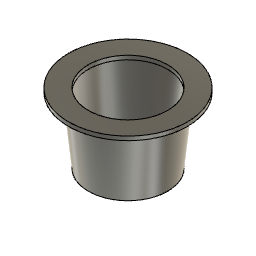
strong plant pot (Autodesk Fusion 360 design; units mm, degrees)
Autodesk Fusion 360 part; units mm, degrees
sketch "Sketch1" plane through (0, 0, 0) normal (0, 0, 1) x (1, 0, 0)
  circle A0 centre (0, 0) radius 30
  circle A1 centre (0, 0) radius 25
  dimension "d1" = 60
  dimension "d7" = 50
  constraint coincident A0.centre A1.centre
  constraint concentric A0 A1
  measures "d1" diameter of A0
  measures "d7" diameter of A1
ref_plane "WorkPlane1" through (0, 0, 50) normal (0, 0, 1) x (1, 0, 0)
ref_plane "WorkPlane2" through (0, 0, 50) normal (0, 0, 1) x (1, 0, 0)
ref_plane "WorkPlane3" through (0, 0, 50) normal (0, 0, 1) x (1, 0, 0)
sketch "Sketch7" plane through (0, 0, 50) normal (0, 0, 1) x (1, 0, 0)
  circle A0 centre (0, 0) radius 35
  circle A1 centre (0, 0) radius 30
  dimension "d6" = 70
  dimension "d8" = 60
  constraint coincident A0.centre A1.centre
  measures "d6" diameter of A0
  measures "d8" diameter of A1
loft "Loft1" add profiles "Sketch7", "Sketch1" section 1 section 2
sketch "Sketch8" plane through (0, 0, 50) normal (0, 0, 1) x (-1, 0, 0)
  circle A0 centre (0, 0) radius 35
  circle A1 centre (0, 0) radius 30
  dimension "d9" = 60
  constraint coincident A0.centre A1.centre
  measures "d9" diameter of A1
sketch "Sketch9" plane through (0, 0, 0) normal (0, 0, -1) x (1, 0, 0)
  circle A0 centre (0, 0) radius 30
  circle A1 centre (0, 0) radius 25
  constraint coincident A0.centre A1.centre
loft "Loft2" cut profiles "Sketch8", "Sketch9" section 1 contours A1 section 2 contours A1
sketch "Sketch11" plane through (0, 0, 50) normal (0, 0, 1) x (-1, 0, 0)
  circle A0 centre (0, 0) radius 30
  circle A1 centre (0, 0) radius 35
  circle A2 centre (0, 0) radius 30
  circle A3 centre (0, 0) radius 45
  dimension "d14" = 90
  constraint coincident A0.centre A1.centre
  constraint concentric A2 A3
  measures "d14" diameter of A3
extrude "Extrude2" add sketch "Sketch11" along normal blind 3 contours A1 | A3
sketch "Sketch12" plane through (0, 0, 0) normal (0, 0, -1) x (1, 0, 0)
  circle A0 centre (0, 0) radius 25
  circle A1 centre (0, 0) radius 30
  circle A2 centre (0, 0) radius 25
  circle A3 centre (0, 0) radius 20
  dimension "d17" = 40
  constraint coincident A0.centre A1.centre
  constraint concentric A2 A3
  measures "d17" diameter of A3
extrude "Extrude3" add sketch "Sketch12" against normal blind 5 contours A0 A2
sketch "Sketch10" plane through (0, 0, 50) normal (0, 0, 1) x (-1, 0, 0)
  circle A0 centre (0, 0) radius 30
  circle A1 centre (0, 0) radius 35
  circle A2 centre (0, 0) radius 45
  circle A3 centre (0, 0) radius 35
  dimension "d10" = 90
  dimension "d13" = 70
  constraint coincident A0.centre A1.centre
  measures "d10" diameter of A2
  measures "d13" diameter of A3
extrude "Extrude1" [rolled back] along distance 3 taper angle 0
